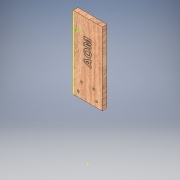
# Autodesk Inventor part: ARM extension 6 mm with drawing
Saved by Autodesk Inventor 2018 (Build 220112000, 112)
## iProperties
Created: 2018-03-26
Part Number: ARM extension 6 mm with drawing
Material: Wood (Birch)
Document SubType Name: Modeling
Designer: omara
Density: 0.55 g/cm^3
Appearance: Birch - Natural Polished
Author: omara
Autodesk Inventor part; units mm, degrees
ref_plane "YZ Plane" through (0, 0, 0) normal (1, 0, 0) x (0, 1, 0)
ref_plane "XZ Plane" through (0, 0, 0) normal (0, 1, 0) x (-1, 0, 0)
ref_plane "XY Plane" through (0, 0, 0) normal (0, 0, 1) x (1, 0, 0)
sketch "Sketch4" plane through (0, 0, 0) normal (0, 0, 1) x (1, 0, 0)
  line L0 (7.5655, 305.2492) -> (7.5655, 174.3515)
  line L1 (7.5655, 174.2904) -> (-7.4345, 179.5716)
  line L2 (-7.4345, 179.5716) -> (-7.4345, 184.4493)
  line L3 (-7.4345, 184.4493) -> (7.5655, 189.7183)
  line L4 (7.5655, 189.7183) -> (7.5655, 184.9383)
  line L5 (7.5655, 184.9383) -> (5.5851, 184.3882)
  line L6 (5.5851, 184.3882) -> (5.5851, 179.6082)
  line L7 (5.5851, 179.6082) -> (7.5655, 179.0214)
  line L8 (7.5655, 179.0214) -> (7.5655, 174.2904)
  line L9 (7.0888, 174.975) -> (7.0888, 178.7158)
  line L10 (7.0888, 178.7158) -> (5.1083, 179.2537)
  line L11 (5.1083, 179.2537) -> (5.1083, 184.7183)
  line L12 (5.1083, 184.7183) -> (7.0888, 185.2928)
  line L13 (7.0888, 185.2928) -> (7.0888, 189.0337)
  line L14 (7.0888, 189.0337) -> (-6.921, 184.0826)
  line L15 (-6.921, 184.0826) -> (-6.921, 179.9261)
  line L16 (-6.921, 179.9261) -> (7.0888, 174.975)
  line L17 (2.9201, 179.9016) -> (-4.3782, 182.0043)
  line L18 (-4.3782, 182.0043) -> (2.9201, 184.1437)
  line L19 (2.9201, 184.1437) -> (2.9201, 179.9016)
  line L20 (2.4433, 180.4762) -> (2.4433, 183.508)
  line L21 (2.4433, 183.508) -> (-1.7499, 182.2977)
  spline S0 degree 2 poles (-1.7499, 182.2977) (-2.2144, 182.1632) (-2.9112, 182.0288) (-3.2413, 182.0043) knots 0 0 0 1 2 2 2
  spline S1 degree 2 poles (-3.2413, 182.0043) (-2.8868, 181.9676) (-2.1655, 181.8209) (-1.7743, 181.7109) knots 0 0 0 1 2 2 2
  line L22 (-1.7743, 181.7109) -> (2.4433, 180.4762)
  spline S2 degree 2 poles (0.0717, 190.5495) (-3.5836, 190.5495) (-7.8257, 194.7427) (-7.8257, 198.3491) knots 0 0 0 1 2 2 2
  spline S3 degree 2 poles (-7.8257, 198.3491) (-7.8257, 201.9554) (-3.5836, 206.1363) (0.0717, 206.1363) knots 0 0 0 1 2 2 2
  spline S4 degree 2 poles (0.0717, 206.1363) (3.7391, 206.1363) (7.9812, 201.9554) (7.9812, 198.3491) knots 0 0 0 1 2 2 2
  spline S5 degree 2 poles (7.9812, 198.3491) (7.9812, 194.7427) (3.7269, 190.5495) (0.0717, 190.5495) knots 0 0 0 1 2 2 2
  spline S6 degree 2 poles (0.0717, 191.063) (3.4946, 191.063) (7.5044, 194.975) (7.5044, 198.3368) knots 0 0 0 1 2 2 2
  spline S7 degree 2 poles (7.5044, 198.3368) (7.5044, 201.6987) (3.4946, 205.6107) (0.0717, 205.6107) knots 0 0 0 1 2 2 2
  spline S8 degree 2 poles (0.0717, 205.6107) (-3.3636, 205.6107) (-7.3733, 201.6865) (-7.3733, 198.3368) knots 0 0 0 1 2 2 2
  spline S9 degree 2 poles (-7.3733, 198.3368) (-7.3733, 194.975) (-3.3636, 191.063) (0.0717, 191.063) knots 0 0 0 1 2 2 2
  spline S10 degree 2 poles (0.0717, 194.8894) (-2.3122, 194.8894) (-4.5371, 196.5642) (-4.5371, 198.3491) knots 0 0 0 1 2 2 2
  spline S11 degree 2 poles (-4.5371, 198.3491) (-4.5371, 200.1339) (-2.3122, 201.7965) (0.0717, 201.7965) knots 0 0 0 1 2 2 2
  spline S12 degree 2 poles (0.0717, 201.7965) (2.4677, 201.7965) (4.6805, 200.1339) (4.6805, 198.3491) knots 0 0 0 1 2 2 2
  spline S13 degree 2 poles (4.6805, 198.3491) (4.6805, 196.5642) (2.4555, 194.8894) (0.0717, 194.8894) knots 0 0 0 1 2 2 2
  spline S14 degree 2 poles (0.0717, 195.4028) (2.211, 195.4028) (4.2037, 196.8209) (4.2037, 198.3491) knots 0 0 0 1 2 2 2
  spline S15 degree 2 poles (4.2037, 198.3491) (4.2037, 199.865) (2.211, 201.2708) (0.0717, 201.2708) knots 0 0 0 1 2 2 2
  spline S16 degree 2 poles (0.0717, 201.2708) (-2.0677, 201.2708) (-4.0604, 199.865) (-4.0604, 198.3491) knots 0 0 0 1 2 2 2
  spline S17 degree 2 poles (-4.0604, 198.3491) (-4.0604, 196.8209) (-2.0677, 195.4028) (0.0717, 195.4028) knots 0 0 0 1 2 2 2
  line L23 (7.5655, 212.7011) -> (7.5655, 208.3368)
  line L24 (7.5655, 208.3368) -> (-7.4345, 208.3368)
  line L25 (-7.4345, 208.3368) -> (-7.4345, 214.2048)
  line L26 (-7.4345, 214.2048) -> (0.0472, 216.283)
  spline S18 degree 2 poles (0.0472, 216.283) (0.1939, 216.3319) (1.2819, 216.5764) (2.2477, 216.7965) knots 0 0 0 1 2 2 2
  spline S19 degree 2 poles (2.2477, 216.7965) (1.5142, 216.9432) (0.3528, 217.1877) (0.0839, 217.2733) knots 0 0 0 1 2 2 2
  line L27 (0.0839, 217.2733) -> (-7.4345, 219.4004)
  line L28 (-7.4345, 219.4004) -> (-7.4345, 225.2561)
  line L29 (-7.4345, 225.2561) -> (7.5655, 225.2561)
  line L30 (7.5655, 225.2561) -> (7.5655, 220.9407)
  line L31 (7.5655, 220.9407) -> (0.1817, 220.9407)
  spline S20 degree 2 poles (0.1817, 220.9407) (-0.3195, 220.9407) (-2.1655, 221.0263) (-3.2046, 221.0874) knots 0 0 0 1 2 2 2
  spline S21 degree 2 poles (-3.2046, 221.0874) (-1.6765, 220.7574) (0.035, 220.3906) (0.2306, 220.3417) knots 0 0 0 1 2 2 2
  line L32 (0.2306, 220.3417) -> (7.5655, 218.4835)
  line L33 (7.5655, 218.4835) -> (7.5655, 215.1217)
  line L34 (7.5655, 215.1217) -> (0.3895, 213.2513)
  spline S22 degree 2 poles (0.3895, 213.2513) (-0.1362, 213.1046) (-1.9821, 212.7378) (-3.3024, 212.5055) knots 0 0 0 1 2 2 2
  spline S23 degree 2 poles (-3.3024, 212.5055) (-1.8966, 212.5911) (0.0472, 212.7011) (0.3284, 212.7011) knots 0 0 0 1 2 2 2
  line L35 (0.3284, 212.7011) -> (7.5655, 212.7011)
  line L36 (-6.921, 219.7794) -> (3.5435, 216.7965)
  line L37 (3.5435, 216.7965) -> (-6.921, 213.8258)
  line L38 (-6.921, 213.8258) -> (-6.921, 208.8503)
  line L39 (-6.921, 208.8503) -> (7.0888, 208.8503)
  line L40 (7.0888, 208.8503) -> (7.0888, 212.1877)
  line L41 (7.0888, 212.1877) -> (-4.2315, 212.1877)
  line L42 (-4.2315, 212.1877) -> (-4.2315, 212.6033)
  line L43 (-4.2315, 212.6033) -> (7.0888, 215.5006)
  line L44 (7.0888, 215.5006) -> (7.0888, 218.0923)
  line L45 (7.0888, 218.0923) -> (-4.2315, 220.9407)
  line L46 (-4.2315, 220.9407) -> (-4.2315, 221.4542)
  line L47 (-4.2315, 221.4542) -> (7.0888, 221.4542)
  line L48 (7.0888, 221.4542) -> (7.0888, 224.7427)
  line L49 (7.0888, 224.7427) -> (-6.921, 224.7427)
  line L50 (-6.921, 224.7427) -> (-6.921, 219.7794)
  point P0 (0, 0)
  constraints: 2 end point, 2 vertical
sketch "Sketch2" plane through (0, 0, 0) normal (0, 0, 1) x (1, 0, 0)
  circle A0 centre (12.5029, 140.4545) radius 2
  line L0 (0.0029, 135.929) -> (0.0029, 127.4079) construction
  line L1 (-18.9761, 149.4259) -> (-18.9761, 119.8067)
  line L2 (-34.3555, 140.9765) -> (34.7909, 140.9765)
  line L3 (0.0029, 127.4079) -> (0.0029, 126.5093)
  line L4 (-15.0758, 140.9765) -> (-15.0758, 120.9765)
  line L5 (-15.0758, 120.9765) -> (-22.5601, 120.9765)
  line L6 (0.0029, 126.7136) -> (0.0029, 116.7135)
  circle A1 centre (-12.4971, 140.4545) radius 2
  line L7 (19.0411, 120.9644) -> (-4.2564, 120.9644)
  circle A2 centre (19, 120.9644) radius 2
  circle A3 centre (-18.9943, 120.9644) radius 2
  line L8 (30, 110) -> (0, 110)
  line L9 (0, 110) -> (0, 260)
  line L10 (0, 260) -> (30, 260)
  line L11 (30, 260) -> (30, 110)
  line L12 (-30, 110) -> (0, 110)
  line L13 (0, 260) -> (-30, 260)
  line L14 (-30, 260) -> (-30, 110)
  point P0 (0, 0)
  dimension "d32" = 20
  dimension "d41" = 25
  dimension "d60" = 4
  dimension "d61" = 150
  constraints: 30 end point, 5 vertical, 4 centre point, 4 horizontal, 4 symmetric about line, 3 point on line, 2 parallel, 1 perpendicular, 2 other
  measures "d32" distance of L4.start L4.end
  measures "d41" distance of A0.centre A1.centre
  measures "d60" diameter of A2
  measures "d61" distance of L8.end L9.end
extrude "Extrusion5" add sketch "Sketch2" along normal blind 10 contours A0 L2 L11 L8 L9 | A0 L2 L9 L10 L11 | L9 L12 L14 L2 L1 A3 L5 L4 A1 | L2 A1 L14 L13 L9 | L4 L5 A3 L1 L2
extrude "Extrusion6" cut sketch "Sketch4" along normal through all contours L0 L5 L6 L7 L8 L1 L2 L3 | S4 S5 L0 | L0 S5 S2 S3 S4 | L0 L31 S20 S21 L32 L34 S22 S23 L35 L24 L25 L26 S18 S19 L27 L28 L29 | L17 L18 L19 | S10 S11 S12 S13
sketch "Sketch5" plane through (0, 0, 10) normal (0, 0, 1) x (1, 0, 0)
  line L0 (-30, 260) -> (-30, 110) projected
  line L1 (-30, 230) -> (-13.9566, 230)
  point P0 (0, 0)
  constraints: 2 end point, 1 perpendicular, 1 point on line
body "Solid5"
